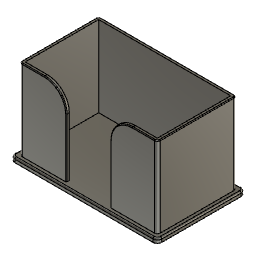
Credit Card storage box v3 (Autodesk Fusion 360 design; units mm, degrees)
Autodesk Fusion 360 part; units mm, degrees
sketch "Sketch1" plane through (0, 0, 0) normal (0, 0, 1) x (1, 0, 0)
  line L0 (0, 0) -> (90, 0)
  line L1 (90, 0) -> (90, 50)
  line L2 (90, 50) -> (0, 50)
  line L3 (0, 50) -> (0, 0)
  line L4 (-2, -2) -> (92, -2)
  line L5 (92, -2) -> (92, 52)
  line L6 (92, 52) -> (-2, 52)
  line L7 (-2, 52) -> (-2, -2)
  line L8 (-5, -5) -> (95, -5)
  line L9 (95, -5) -> (95, 55)
  line L10 (95, 55) -> (-5, 55)
  line L11 (-5, 55) -> (-5, -5)
  line L12 (30, 0) -> (60, 0)
  line L13 (60, 0) -> (60, -2)
  line L14 (60, -2) -> (30, -2)
  line L15 (30, -2) -> (30, 0)
  dimension "d1" = 90
  dimension "d2" = 50
  dimension "d3" = 2
  dimension "d4" = 5
  dimension "d5" = 30
  constraint horizontal L0
  constraint vertical L1
  constraint horizontal L2
  constraint vertical L3
  constraint coincident L0.start L3.end
  constraint horizontal L12
  constraint vertical L13
  constraint horizontal L14
  constraint vertical L15
  constraint coincident L0 L12.start
  constraint midpoint L0 L12
  measures "d1" distance of L0.start L0.end
  measures "d2" distance of L0.start L2.end
  measures "d5" distance of L12.start L12.end
extrude "Extrude1" add sketch "Sketch1" along normal blind 55 contours L0 L1 L2 L3 L4 L5 L6 L7 L13 L15
extrude "Extrude2" add sketch "Sketch1" against normal blind 3 contours L0 L1 L2 L3 L12 | L0 L1 L2 L3 L4 L5 L6 L7 L13 L15 | L0 L4 L12 L13 L14 L15 | L8 L9 L10 L11
fillet "Fillet1" radius 15 2 edges at (30, -1, 55) (60, -1, 55)
fillet "Fillet2" radius 3 4 edges at (-5, -5, -1.5) (95, -5, -1.5) (95, 55, -1.5) (-5, 55, -1.5)
fillet "Fillet3" radius 2 4 edges at (92, -2, 27.5) (92, 52, 27.5) (-2, -2, 27.5) (-2, 52, 27.5)
fillet "Fillet4" radius 0.5 13 edges at (30, -2, 20) (25.6066, -2, 50.6066) (7.5, -2, 55) (-1.4142, -1.4142, 55) (-2, 25, 55) (-1.4142, 51.4142, 55) (45, 52, 55) (91.4142, 51.4142, 55) (92, 25, 55) (91.4142, -1.4142, 55) (82.5, -2, 55) (64.3934, -2, 50.6066) (60, -2, 20)
fillet "Fillet5" radius 1 8 edges at (94.1213, -4.1213, 0) (95, 25, 0) (94.1213, 54.1213, 0) (45, 55, 0) (-4.1213, 54.1213, 0) (-5, 25, 0) (-4.1213, -4.1213, 0) (45, -5, 0)
equation "d1 = base_width"
equation "d2 = base_depth"
equation "d3 = wall_thickness"
equation "d4 = wall_thickness + base_overhang"
equation "d5 = base_width / 3"
equation "d6 = wall_height"
equation "d8 = -( wall_thickness + 1 mm )"
equation "base_width = 90 mm"
equation "base_depth = 50 mm"
equation "wall_height = 55 mm"
equation "wall_thickness = 2 mm"
equation "base_overhang = 3 mm"
